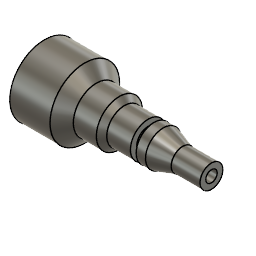
CNC TURNING (Autodesk Fusion 360 design; units mm, degrees)
part number: 2026-06-22-22-29-52-944
Autodesk Fusion 360 part; units mm, degrees
sketch "Sketch1" plane through (0, 0, 0) normal (0, 0, 1) x (1, 0, 0)
  line L0 (0, 0) -> (0, 60.4496)
  line L1 (0, 60.4496) -> (70, 60.4496)
  line L2 (70, 60.4496) -> (90, 40)
  line L3 (90, 40) -> (130, 40)
  line L4 (130, 40) -> (138.9297, 30.8696)
  line L5 (138.9297, 30.8696) -> (163.3358, 30.8696)
  line L6 (200, 0) -> (0, 0)
  line L7 (260, 0) -> (200, 0)
  line L8 (180, 20) -> (190, 20)
  line L9 (190, 20) -> (190, 30.8696)
  line L10 (190, 30.8696) -> (206.2856, 30.8696)
  line L11 (206.2856, 30.8696) -> (240, 20)
  line L12 (240, 20) -> (284.6944, 20)
  line L13 (284.6944, 20) -> (290, 20)
  line L14 (260, 0) -> (290, 0)
  line L15 (290, 0) -> (290, 20)
  line L16 (180, 20) -> (180, 30.8696)
  line L17 (180, 30.8696) -> (163.3358, 30.8696)
  constraint coincident L0.start L6.end
  constraint vertical L0
  constraint perpendicular L0 L1
  constraint parallel L1 L3
  constraint parallel L2 L4
  constraint parallel L3 L5
  constraint perpendicular L0 L6
  constraint parallel L5 L8
  constraint perpendicular L5 L9
  constraint perpendicular L9 L10
  constraint perpendicular L9 L12
  constraint parallel L12 L13
  constraint parallel L7 L14
  constraint perpendicular L13 L15
  constraint perpendicular L8 L16
  constraint perpendicular L16 L17
revolve "Revolve1" add sketch "Sketch1" angle 360 about axis through (260, 0, 0) along (-1, 0, 0)
hole "Hole1" at (290, 0, 0) direction (-1, 0, 0) diameter 20 depth 20 tip angle 118
